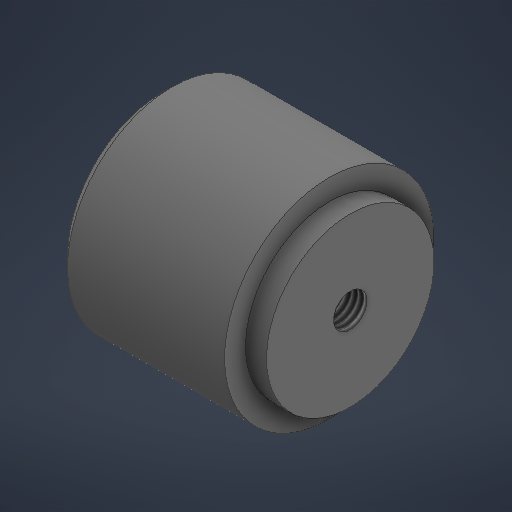
# Autodesk Inventor part: üllő
Saved by Autodesk Inventor 2025 (Build 290162010, 162A)
## iProperties
Created: 2025-02-13
Part Number: üllő
Material: Generic
Document SubType Name: Modeling
Designer: petruska.milan
Density: 1 g/cm^3
Appearance: Default
Author: petruska.milan
Autodesk Inventor part; units mm, degrees
ref_plane "YZ Plane" through (0, 0, 0) normal (1, 0, 0) x (0, 1, 0)
ref_plane "XZ Plane" through (0, 0, 0) normal (0, 1, 0) x (-1, 0, 0)
ref_plane "XY Plane" through (0, 0, 0) normal (0, 0, 1) x (1, 0, 0)
sketch "Sketch1" plane through (0, 0, 0) normal (0, 0, 1) x (1, 0, 0)
  line L0 (0, 0) -> (18, 0)
  line L1 (18, 0) -> (18, 10)
  line L2 (18, 10) -> (0, 10)
  line L3 (0, 10) -> (0, 0)
  line L4 (18, 0) -> (16, 0)
  line L5 (16, 0) -> (16, 8)
  line L6 (16, 8) -> (18, 8)
  line L7 (18, 8) -> (18, 0)
  line L8 (16, 8) -> (16, 10)
  dimension "d0" = 18
  dimension "d1" = 10
  dimension "d2" = 2
  dimension "d3" = 8
  constraints: 18 end point, 4 parallel, 3 perpendicular, 2 horizontal, 1 point on line
  measures "d0" distance of L2.end L1.end
  measures "d1" distance of L1.end L0.end
  measures "d2" distance of L5.end L6.end
  measures "d3" distance of L4.end L5.end
revolve "Revolution1" add sketch "Sketch1" angle 360 about axis through (0, 0, 0) along (1, 0, 0) contours L3 L2 L8 L5 L0 | L5 L6 L1 L0
chamfer "Chamfer1" distance 1 angle 45 1 edges at (0, -10, 0)
sketch "Sketch2" plane through (18, 0, 0) normal (1, 0, 0) x (0, 0, -1)
  point P0 (0, 0)
  point P1 (0, 0)
  constraints: 1 coincident
hole "Hole1" at (18, 0, 0) direction (-1, 0, 0) diameter 3.2 depth 14 tip angle 118
thread "Thread1" size "M3.5x0.6" class "6H" standard "ANSI Metric M Profile" length 10.5
body "Solid1"
